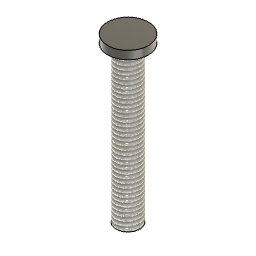
Stepper_screw (Autodesk Fusion 360 design; units mm, degrees)
Autodesk Fusion 360 part; units mm, degrees
sketch "Sketch1" plane through (0, 0, 0) normal (0, 0, 1) x (1, 0, 0)
  circle A0 centre (0, 0) radius 1.5
  dimension "d1" = 3
  constraint coincident A0.centre origin
  measures "d1" diameter of A0
extrude "Extrude1" add sketch "Sketch1" along normal blind 19 makes body 1
sketch "Sketch2" plane through (0, 0, 19) normal (0, 0, 1) x (-1, 0, 0)
  circle A0 centre (0, 0) radius 1.5
  circle A1 centre (0, 0) radius 2.5
  dimension "d4" = 5
  constraint concentric A0 A1
  measures "d4" diameter of A1
extrude "Extrude2" add sketch "Sketch2" along normal blind 1 separate body makes body 2
extrude "Extrude3" add 1 faces at (0.567, -0.5383, 19) along direction (0, 0, 1) blind 1 on bodies 1 bodies 1 2
thread "Thread1" "ISO Metric profile 3.0 M3x0.5 6g" major diameter 2.927 minor diameter 2.3555 pitch 0.5 angle 60 resizes the face on face at (1.4981, -0.0748, 6.3333) on bodies 1
